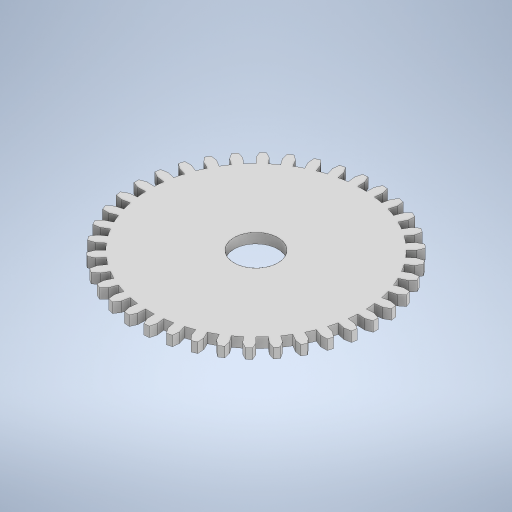
# Autodesk Inventor part: M3_38
Saved by Autodesk Inventor 2024.1 (Build 281209000, 209)
## iProperties
Created: 2024-04-01
Part Number: M3_38
Material: 一般
Document SubType Name: Modeling
Designer: hibik
Density: 1 g/cm^3
Appearance: 既定
Author: hibik
Autodesk Inventor part; units mm, degrees
ref_plane "YZ Plane" through (0, 0, 0) normal (1, 0, 0) x (0, 1, 0)
ref_plane "XZ Plane" through (0, 0, 0) normal (0, 1, 0) x (-1, 0, 0)
ref_plane "XY Plane" through (0, 0, 0) normal (0, 0, 1) x (1, 0, 0)
sketch "スケッチ1" plane through (0, 0, 0) normal (0, 1, 0) x (-1, 0, 0)
  circle A0 centre (0, 0) radius 57 construction
  circle A1 centre (0, 0) radius 60 construction
  line L0 (60, 1.2454) -> (60, -1.2454)
  line L1 (60, 1.2454) -> (56.9513, 2.355)
  line L2 (60, -1.2454) -> (56.9513, -2.355)
  line L3 (84, 0) -> (-84, 0) projected
  circle A2 centre (0, 0) radius 53.25
  line L4 (56.9513, -2.355) -> (53.2045, -2.2001)
  line L5 (56.9513, 2.355) -> (53.2045, 2.2001)
  line L6 (55.787, 11.6968) -> (52.1168, 10.9272)
  line L7 (58.9767, 11.1041) -> (55.787, 11.6968)
  line L8 (58.9767, 11.1041) -> (59.3867, 8.6473)
  line L9 (59.3867, 8.6473) -> (56.5622, 7.051)
  line L10 (56.5622, 7.051) -> (52.841, 6.5871)
  line L11 (53.1009, 20.7195) -> (49.6074, 19.3563)
  line L12 (56.3447, 20.6599) -> (53.1009, 20.7195)
  line L13 (56.3447, 20.6599) -> (57.1534, 18.3041)
  line L14 (57.1534, 18.3041) -> (54.6302, 16.2647)
  line L15 (54.6302, 16.2647) -> (51.0361, 15.1946)
  line L16 (48.9663, 29.177) -> (45.7449, 27.2575)
  line L17 (52.1757, 29.6521) -> (48.9663, 29.177)
  line L18 (52.1757, 29.6521) -> (53.3612, 27.4616)
  line L19 (53.3612, 27.4616) -> (51.2081, 25.0347)
  line L20 (51.2081, 25.0347) -> (47.8391, 23.3877)
  line L21 (43.4961, 36.8387) -> (40.6345, 34.4151)
  line L22 (46.5835, 37.8355) -> (43.4961, 36.8387)
  line L23 (46.5835, 37.8355) -> (48.1134, 35.87)
  line L24 (48.1134, 35.87) -> (46.3891, 33.1218)
  line L25 (46.3891, 33.1218) -> (43.3372, 30.9427)
  line L26 (36.8395, 43.4955) -> (34.4158, 40.6339)
  line L27 (39.7206, 44.9869) -> (36.8395, 43.4955)
  line L28 (39.7206, 44.9869) -> (41.5531, 43.3)
  line L29 (41.5531, 43.3) -> (40.3047, 40.3055)
  line L30 (40.3047, 40.3055) -> (37.6531, 37.6538)
  line L31 (29.1779, 48.9658) -> (27.2583, 45.7444)
  line L32 (31.7743, 50.9111) -> (29.1779, 48.9658)
  line L33 (31.7743, 50.9111) -> (33.8595, 49.5488)
  line L34 (33.8595, 49.5488) -> (33.121, 46.3897)
  line L35 (33.121, 46.3897) -> (30.9419, 43.3377)
  line L36 (20.7204, 53.1005) -> (19.3573, 49.607)
  line L37 (22.9612, 55.4467) -> (20.7204, 53.1005)
  line L38 (22.9612, 55.4467) -> (25.2422, 54.4461)
  line L39 (25.2422, 54.4461) -> (25.0337, 51.2085)
  line L40 (25.0337, 51.2085) -> (23.3868, 47.8395)
  line L41 (11.6978, 55.7868) -> (10.9282, 52.1166)
  line L42 (13.5219, 58.4697) -> (11.6978, 55.7868)
  line L43 (13.5219, 58.4697) -> (15.9364, 57.8583)
  line L44 (15.9364, 57.8583) -> (16.2637, 54.6305)
  line L45 (16.2637, 54.6305) -> (15.1937, 51.0364)
  line L46 (2.356, 56.9513) -> (2.201, 53.2045)
  line L47 (3.7136, 59.8979) -> (2.356, 56.9513)
  line L48 (3.7136, 59.8979) -> (6.1959, 59.6922)
  line L49 (6.1959, 59.6922) -> (7.05, 56.5623)
  line L50 (7.05, 56.5623) -> (6.5861, 52.8411)
  line L51 (-7.05, 56.5623) -> (-6.5861, 52.8411)
  line L52 (-6.1959, 59.6922) -> (-7.05, 56.5623)
  line L53 (-6.1959, 59.6922) -> (-3.7136, 59.8979)
  line L54 (-3.7136, 59.8979) -> (-2.356, 56.9513)
  line L55 (-2.356, 56.9513) -> (-2.201, 53.2045)
  line L56 (-16.2637, 54.6305) -> (-15.1937, 51.0364)
  line L57 (-15.9364, 57.8583) -> (-16.2637, 54.6305)
  line L58 (-15.9364, 57.8583) -> (-13.5219, 58.4697)
  line L59 (-13.5219, 58.4697) -> (-11.6978, 55.7868)
  line L60 (-11.6978, 55.7868) -> (-10.9282, 52.1166)
  line L61 (-25.0337, 51.2085) -> (-23.3868, 47.8395)
  line L62 (-25.2422, 54.4461) -> (-25.0337, 51.2085)
  line L63 (-25.2422, 54.4461) -> (-22.9612, 55.4467)
  line L64 (-22.9612, 55.4467) -> (-20.7204, 53.1005)
  line L65 (-20.7204, 53.1005) -> (-19.3573, 49.607)
  line L66 (-33.121, 46.3897) -> (-30.9419, 43.3377)
  line L67 (-33.8595, 49.5488) -> (-33.121, 46.3897)
  line L68 (-33.8595, 49.5488) -> (-31.7743, 50.9111)
  line L69 (-31.7743, 50.9111) -> (-29.1779, 48.9658)
  line L70 (-29.1779, 48.9658) -> (-27.2583, 45.7444)
  line L71 (-40.3047, 40.3055) -> (-37.6531, 37.6538)
  line L72 (-41.5531, 43.3) -> (-40.3047, 40.3055)
  line L73 (-41.5531, 43.3) -> (-39.7206, 44.9869)
  line L74 (-39.7206, 44.9869) -> (-36.8395, 43.4955)
  line L75 (-36.8395, 43.4955) -> (-34.4158, 40.6339)
  line L76 (-46.3891, 33.1218) -> (-43.3372, 30.9427)
  line L77 (-48.1134, 35.87) -> (-46.3891, 33.1218)
  line L78 (-48.1134, 35.87) -> (-46.5835, 37.8355)
  line L79 (-46.5835, 37.8355) -> (-43.4961, 36.8387)
  line L80 (-43.4961, 36.8387) -> (-40.6345, 34.4151)
  line L81 (-51.2081, 25.0347) -> (-47.8391, 23.3877)
  line L82 (-53.3612, 27.4616) -> (-51.2081, 25.0347)
  line L83 (-53.3612, 27.4616) -> (-52.1757, 29.6521)
  line L84 (-52.1757, 29.6521) -> (-48.9663, 29.177)
  line L85 (-48.9663, 29.177) -> (-45.7449, 27.2575)
  line L86 (-54.6302, 16.2647) -> (-51.0361, 15.1946)
  line L87 (-57.1534, 18.3041) -> (-54.6302, 16.2647)
  line L88 (-57.1534, 18.3041) -> (-56.3447, 20.6599)
  line L89 (-56.3447, 20.6599) -> (-53.1009, 20.7195)
  line L90 (-53.1009, 20.7195) -> (-49.6074, 19.3563)
  line L91 (-56.5622, 7.051) -> (-52.841, 6.5871)
  line L92 (-59.3867, 8.6473) -> (-56.5622, 7.051)
  line L93 (-59.3867, 8.6473) -> (-58.9767, 11.1041)
  line L94 (-58.9767, 11.1041) -> (-55.787, 11.6968)
  line L95 (-55.787, 11.6968) -> (-52.1168, 10.9272)
  line L96 (-56.9513, -2.355) -> (-53.2045, -2.2001)
  line L97 (-60, -1.2454) -> (-56.9513, -2.355)
  line L98 (-60, -1.2454) -> (-60, 1.2454)
  line L99 (-60, 1.2454) -> (-56.9513, 2.355)
  line L100 (-56.9513, 2.355) -> (-53.2045, 2.2001)
  line L101 (-55.787, -11.6968) -> (-52.1168, -10.9272)
  line L102 (-58.9767, -11.1041) -> (-55.787, -11.6968)
  line L103 (-58.9767, -11.1041) -> (-59.3867, -8.6473)
  line L104 (-59.3867, -8.6473) -> (-56.5622, -7.051)
  line L105 (-56.5622, -7.051) -> (-52.841, -6.5871)
  line L106 (-53.1009, -20.7195) -> (-49.6074, -19.3563)
  line L107 (-56.3447, -20.6599) -> (-53.1009, -20.7195)
  line L108 (-56.3447, -20.6599) -> (-57.1534, -18.3041)
  line L109 (-57.1534, -18.3041) -> (-54.6302, -16.2647)
  line L110 (-54.6302, -16.2647) -> (-51.0361, -15.1946)
  line L111 (-48.9663, -29.177) -> (-45.7449, -27.2575)
  line L112 (-52.1757, -29.6521) -> (-48.9663, -29.177)
  line L113 (-52.1757, -29.6521) -> (-53.3612, -27.4616)
  line L114 (-53.3612, -27.4616) -> (-51.2081, -25.0347)
  line L115 (-51.2081, -25.0347) -> (-47.8391, -23.3877)
  line L116 (-43.4961, -36.8387) -> (-40.6345, -34.4151)
  line L117 (-46.5835, -37.8355) -> (-43.4961, -36.8387)
  line L118 (-46.5835, -37.8355) -> (-48.1134, -35.87)
  line L119 (-48.1134, -35.87) -> (-46.3891, -33.1218)
  line L120 (-46.3891, -33.1218) -> (-43.3372, -30.9427)
  line L121 (-36.8395, -43.4955) -> (-34.4158, -40.6339)
  line L122 (-39.7206, -44.9869) -> (-36.8395, -43.4955)
  line L123 (-39.7206, -44.9869) -> (-41.5531, -43.3)
  line L124 (-41.5531, -43.3) -> (-40.3047, -40.3055)
  line L125 (-40.3047, -40.3055) -> (-37.6531, -37.6538)
  line L126 (-29.1779, -48.9658) -> (-27.2583, -45.7444)
  line L127 (-31.7743, -50.9111) -> (-29.1779, -48.9658)
  line L128 (-31.7743, -50.9111) -> (-33.8595, -49.5488)
  line L129 (-33.8595, -49.5488) -> (-33.121, -46.3897)
  line L130 (-33.121, -46.3897) -> (-30.9419, -43.3377)
  line L131 (-20.7204, -53.1005) -> (-19.3573, -49.607)
  line L132 (-22.9612, -55.4467) -> (-20.7204, -53.1005)
  line L133 (-22.9612, -55.4467) -> (-25.2422, -54.4461)
  line L134 (-25.2422, -54.4461) -> (-25.0337, -51.2085)
  line L135 (-25.0337, -51.2085) -> (-23.3868, -47.8395)
  line L136 (-11.6978, -55.7868) -> (-10.9282, -52.1166)
  line L137 (-13.5219, -58.4697) -> (-11.6978, -55.7868)
  line L138 (-13.5219, -58.4697) -> (-15.9364, -57.8583)
  line L139 (-15.9364, -57.8583) -> (-16.2637, -54.6305)
  line L140 (-16.2637, -54.6305) -> (-15.1937, -51.0364)
  line L141 (-2.356, -56.9513) -> (-2.201, -53.2045)
  line L142 (-3.7136, -59.8979) -> (-2.356, -56.9513)
  line L143 (-3.7136, -59.8979) -> (-6.1959, -59.6922)
  line L144 (-6.1959, -59.6922) -> (-7.05, -56.5623)
  line L145 (-7.05, -56.5623) -> (-6.5861, -52.8411)
  line L146 (7.05, -56.5623) -> (6.5861, -52.8411)
  line L147 (6.1959, -59.6922) -> (7.05, -56.5623)
  line L148 (6.1959, -59.6922) -> (3.7136, -59.8979)
  line L149 (3.7136, -59.8979) -> (2.356, -56.9513)
  line L150 (2.356, -56.9513) -> (2.201, -53.2045)
  line L151 (16.2637, -54.6305) -> (15.1937, -51.0364)
  line L152 (15.9364, -57.8583) -> (16.2637, -54.6305)
  line L153 (15.9364, -57.8583) -> (13.5219, -58.4697)
  line L154 (13.5219, -58.4697) -> (11.6978, -55.7868)
  line L155 (11.6978, -55.7868) -> (10.9282, -52.1166)
  line L156 (25.0337, -51.2085) -> (23.3868, -47.8395)
  line L157 (25.2422, -54.4461) -> (25.0337, -51.2085)
  line L158 (25.2422, -54.4461) -> (22.9612, -55.4467)
  line L159 (22.9612, -55.4467) -> (20.7204, -53.1005)
  line L160 (20.7204, -53.1005) -> (19.3573, -49.607)
  line L161 (33.121, -46.3897) -> (30.9419, -43.3377)
  line L162 (33.8595, -49.5488) -> (33.121, -46.3897)
  line L163 (33.8595, -49.5488) -> (31.7743, -50.9111)
  line L164 (31.7743, -50.9111) -> (29.1779, -48.9658)
  line L165 (29.1779, -48.9658) -> (27.2583, -45.7444)
  line L166 (40.3047, -40.3055) -> (37.6531, -37.6538)
  line L167 (41.5531, -43.3) -> (40.3047, -40.3055)
  line L168 (41.5531, -43.3) -> (39.7206, -44.9869)
  line L169 (39.7206, -44.9869) -> (36.8395, -43.4955)
  line L170 (36.8395, -43.4955) -> (34.4158, -40.6339)
  line L171 (46.3891, -33.1218) -> (43.3372, -30.9427)
  line L172 (48.1134, -35.87) -> (46.3891, -33.1218)
  line L173 (48.1134, -35.87) -> (46.5835, -37.8355)
  line L174 (46.5835, -37.8355) -> (43.4961, -36.8387)
  line L175 (43.4961, -36.8387) -> (40.6345, -34.4151)
  line L176 (51.2081, -25.0347) -> (47.8391, -23.3877)
  line L177 (53.3612, -27.4616) -> (51.2081, -25.0347)
  line L178 (53.3612, -27.4616) -> (52.1757, -29.6521)
  line L179 (52.1757, -29.6521) -> (48.9663, -29.177)
  line L180 (48.9663, -29.177) -> (45.7449, -27.2575)
  line L181 (54.6302, -16.2647) -> (51.0361, -15.1946)
  line L182 (57.1534, -18.3041) -> (54.6302, -16.2647)
  line L183 (57.1534, -18.3041) -> (56.3447, -20.6599)
  line L184 (56.3447, -20.6599) -> (53.1009, -20.7195)
  line L185 (53.1009, -20.7195) -> (49.6074, -19.3563)
  line L186 (56.5622, -7.051) -> (52.841, -6.5871)
  line L187 (59.3867, -8.6473) -> (56.5622, -7.051)
  line L188 (59.3867, -8.6473) -> (58.9767, -11.1041)
  line L189 (58.9767, -11.1041) -> (55.787, -11.6968)
  line L190 (55.787, -11.6968) -> (52.1168, -10.9272)
  circle A3 centre (0, 0) radius 11
  point P0 (60, 0)
  point P1 (59.1817, 9.8757)
  point P2 (56.749, 19.482)
  point P3 (52.7684, 28.5568)
  point P4 (47.3484, 36.8528)
  point P5 (40.6369, 44.1434)
  point P6 (32.8169, 50.23)
  point P7 (24.1017, 54.9464)
  point P8 (14.7291, 58.164)
  point P9 (4.9548, 59.7951)
  point P10 (-4.9548, 59.7951)
  point P11 (-14.7291, 58.164)
  point P12 (-24.1017, 54.9464)
  point P13 (-32.8169, 50.23)
  point P14 (-40.6369, 44.1434)
  point P15 (-47.3484, 36.8528)
  point P16 (-52.7684, 28.5568)
  point P17 (-56.749, 19.482)
  point P18 (-59.1817, 9.8757)
  point P19 (-60, 0)
  point P20 (-59.1817, -9.8757)
  point P21 (-56.749, -19.482)
  point P22 (-52.7684, -28.5568)
  point P23 (-47.3484, -36.8528)
  point P24 (-40.6369, -44.1434)
  point P25 (-32.8169, -50.23)
  point P26 (-24.1017, -54.9464)
  point P27 (-14.7291, -58.164)
  point P28 (-4.9548, -59.7951)
  point P29 (4.9548, -59.7951)
  point P30 (14.7291, -58.164)
  point P31 (24.1017, -54.9464)
  point P32 (32.8169, -50.23)
  point P33 (40.6369, -44.1434)
  point P34 (47.3484, -36.8528)
  point P35 (52.7684, -28.5568)
  point P36 (56.749, -19.482)
  point P37 (59.1817, -9.8757)
  point P38 (-43.3372, -30.9427)
  point P39 (-40.6345, -34.4151)
  point P40 (-37.6531, -37.6538)
  point P41 (-34.4158, -40.6339)
  point P42 (-30.9419, -43.3377)
  point P43 (-19.3573, -49.607)
  point P44 (-15.1937, -51.0364)
  point P45 (-10.9282, -52.1166)
  point P46 (-6.5861, -52.8411)
  point P47 (-2.201, -53.2045)
  point P48 (2.201, -53.2045)
  point P49 (10.9282, -52.1166)
  point P50 (15.1937, -51.0364)
  point P51 (19.3573, -49.607)
  point P52 (23.3868, -47.8395)
  point P53 (27.2583, -45.7444)
  point P54 (30.9419, -43.3377)
  point P55 (34.4158, -40.6339)
  point P56 (37.6531, -37.6538)
  point P57 (40.6345, -34.4151)
  point P58 (43.3372, -30.9427)
  point P59 (45.7449, -27.2575)
  point P60 (47.8391, -23.3877)
  point P61 (49.6074, -19.3563)
  point P62 (51.0361, -15.1946)
  point P63 (52.1168, -10.9272)
  point P64 (52.841, -6.5871)
  point P65 (52.841, 6.5871)
  point P66 (52.1168, 10.9272)
  point P67 (49.6074, 19.3563)
  point P68 (45.7449, 27.2575)
  point P69 (40.6345, 34.4151)
  point P70 (37.6531, 37.6538)
  point P71 (34.4158, 40.6339)
  point P72 (27.2583, 45.7444)
  point P73 (19.3573, 49.607)
  point P74 (15.1937, 51.0364)
  point P75 (10.9282, 52.1166)
  point P76 (6.5861, 52.8411)
  point P77 (2.201, 53.2045)
  point P78 (-2.201, 53.2045)
  point P79 (-6.5861, 52.8411)
  point P80 (-10.9282, 52.1166)
  point P81 (-15.1937, 51.0364)
  point P82 (-19.3573, 49.607)
  point P83 (-23.3868, 47.8395)
  point P84 (-27.2583, 45.7444)
  point P85 (-30.9419, 43.3377)
  point P86 (-34.4158, 40.6339)
  point P87 (-37.6531, 37.6538)
  point P88 (-43.3372, 30.9427)
  point P89 (-45.7449, 27.2575)
  point P90 (-47.8391, 23.3877)
  point P91 (-49.6074, 19.3563)
  point P92 (-51.0361, 15.1946)
  point P93 (-52.1168, 10.9272)
  point P94 (-52.841, -6.5871)
  point P95 (-52.1168, -10.9272)
  point P96 (-51.0361, -15.1946)
  point P97 (-49.6074, -19.3563)
  point P98 (-47.8391, -23.3877)
  dimension "d5" = 106.5
  dimension "d0" = 114
  dimension "d1" = 120
  dimension "d3" = 20
  dimension "d4" = 20
  dimension "d14" = 4.71
  dimension "d18" = 360
  dimension "d24" = 22
  constraints: 380 end point, 77 point on line, 6 coincident, 3 centre point, 2 point on circle, 1 midpoint, 1 tangent, 1 vertical, 496 other
  measures "d0" diameter of A0
  measures "d1" diameter of A1
  measures "d3" angle of L3 L1
  measures "d4" angle of L3 L2
  measures "d14" distance of L2.end L1.end
  measures "d24" diameter of A3
extrude "押し出し1" add sketch "スケッチ1" along normal blind 5 contours L0 L3 A2 L5 L1 | L0 L2 L4 A2 L3 | A2 L3 A3 | L3 A3 A2 | A2 L6 L7 L8 L9 L10 | L186 L187 L188 L189 L190 A2 | A2 L96 L97 L98 L3 | L3 L98 L99 L100 A2 | A2 L11 L12 L13 L14 L15 | L181 L182 L183 L184 L185 A2 | L91 L92 L93 L94 L95 A2 | A2 L101 L102 L103 L104 L105 | A2 L16 L17 L18 L19 L20 | L176 L177 L178 L179 L180 A2 | L86 L87 L88 L89 L90 A2 | A2 L106 L107 L108 L109 L110 | A2 L21 L22 L23 L24 L25 | L171 L172 L173 L174 L175 A2 | L81 L82 L83 L84 L85 A2 | A2 L111 L112 L113 L114 L115 | A2 L26 L27 L28 L29 L30 | L166 L167 L168 L169 L170 A2 | L76 L77 L78 L79 L80 A2 | A2 L116 L117 L118 L119 L120 | A2 L31 L32 L33 L34 L35 | L161 L162 L163 L164 L165 A2 | L71 L72 L73 L74 L75 A2 | A2 L121 L122 L123 L124 L125 | A2 L36 L37 L38 L39 L40 | L156 L157 L158 L159 L160 A2 | L66 L67 L68 L69 L70 A2 | A2 L126 L127 L128 L129 L130 | A2 L41 L42 L43 L44 L45 | L151 L152 L153 L154 L155 A2 | L61 L62 L63 L64 L65 A2 | A2 L131 L132 L133 L134 L135 | A2 L46 L47 L48 L49 L50 | L146 L147 L148 L149 L150 A2 | L56 L57 L58 L59 L60 A2 | A2 L136 L137 L138 L139 L140 | A2 L51 L52 L53 L54 L55 | L141 L142 L143 L144 L145 A2
